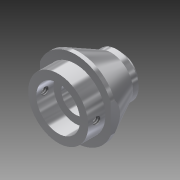
# Autodesk Inventor part: Pneumatic Connector -Actuator Side
Saved by Autodesk Inventor 2013 (Build 170138000, 138)
## iProperties
Created: 2013-06-08
Part Number: Pneumatic Connector -Actuator Side
Material: Generic
Document SubType Name: Modeling
Designer: mvarma
Density: 1 g/cm^3
Author: mvarma
Autodesk Inventor part; units mm, degrees
ref_plane "YZ Plane" through (0, 0, 0) normal (1, 0, 0) x (0, 1, 0)
ref_plane "XZ Plane" through (0, 0, 0) normal (0, 1, 0) x (-1, 0, 0)
ref_plane "XY Plane" through (0, 0, 0) normal (0, 0, 1) x (1, 0, 0)
sketch "Sketch1" plane through (0, 0, 0) normal (0, 0, 1) x (1, 0, 0)
  arc A0 (-1.508, 2.794) -> (-1.508, -2.794) centre (0, 0) ccw
  line L0 (-3.175, 0) -> (0, 0) construction
  line L1 (0, 0) -> (3.175, 0) construction
  line L2 (-1.508, 2.794) -> (1.508, 2.794)
  line L3 (-1.508, -2.794) -> (1.508, -2.794)
  arc A1 (1.508, 2.794) -> (-1.508, 2.794) centre (0, 0) ccw construction
  arc A2 (1.508, -2.794) -> (1.508, 2.794) centre (0, 0) ccw
  arc A3 (-1.508, -2.794) -> (1.508, -2.794) centre (0, 0) ccw construction
  circle A4 centre (0, 0) radius 3.429 construction
  circle A5 centre (0, 0) radius 4.064
  circle A6 centre (0, 0) radius 11.1125
  dimension "d1" = 2.794
  dimension "d2" = 3.175
  dimension "d3" = 6.858
  dimension "d5" = 0.635
  dimension "d6" = 22.225
  constraints: 14 point on circle, 8 end point, 7 centre point, 4 coincident, 2 parallel, 1 collinear, 1 horizontal, 1 other
  measures "d1" distance between parallel lines of L0 L2
  measures "d2" radius of A0
  measures "d3" diameter of A4
  measures "d5" radial gap between concentric circles of A5 A4
  measures "d6" diameter of A6
extrude "Extrusion1" add sketch "Sketch1" along normal blind 3.048 contours A5 | A6
sketch "Sketch2" plane through (0, 0, 3.048) normal (0, 0, 1) x (1, 0, 0)
  circle A0 centre (0, 0) radius 11.1125 projected
  arc A1 (-1.508, 2.794) -> (-1.508, -2.794) centre (0, 0) ccw projected
  constraints: 1 coincident
extrude "Extrusion2" add sketch "Sketch2" along normal blind 3.175
hole "Hole1" at (0, 0, 3.048) direction (0, 0, 1) diameter 3.302 depth 25.4 tip angle 118 thread size "8-32 UNC" class "2B" standard "ANSI Unified Screw Threads"
sketch "Sketch3" plane through (0, 0, 6.223) normal (0, 0, 1) x (1, 0, 0)
  circle A0 centre (0, 0) radius 11.1125 projected
  circle A1 centre (0, 0) radius 3.429
  circle A2 centre (0, 0) radius 4.064
  dimension "d18" = 6.858
  dimension "d19" = 0.635
  constraints: 2 centre point, 2 coincident
  measures "d18" diameter of A1
  measures "d19" radial gap between concentric circles of A2 A1
extrude "Extrusion3" add sketch "Sketch3" along normal blind 7.2961 contours A0
chamfer "Chamfer1" distance 6.35 distance2 12.3571 1 edges at (-11.1125, 0, 0) measured on face at (-10.6125, 0, 0)
sketch "Sketch6" plane through (0, 0, 13.5191) normal (0, 0, 1) x (1, 0, 0)
  circle A0 centre (0, 0) radius 11.1125 projected
  circle A1 centre (0, 0) radius 6.35
  circle A2 centre (0, 0) radius 8.7312
  dimension "d38" = 12.7
  dimension "d52" = 2.3813
  dimension "d53" = 2.3813
  constraints: 2 centre point, 2 coincident
  measures "d38" diameter of A1
  measures "d52" radial gap between concentric circles of A1 A2
  measures "d53" radial gap between concentric circles of A0 A2
extrude "Extrusion5" add sketch "Sketch6" along normal blind 4.9784 contours A2
sketch "Sketch7" plane through (0, 0, 0) normal (1, 0, 0) x (0, 1, 0)
  line L0 (-6.35, 18.4975) -> (6.35, 18.4975) projected
  line L1 (6.35, 13.5191) -> (-6.35, 13.5191) projected
  line L2 (0, 0) -> (0, 13.5191) construction
  line L3 (0, 13.5191) -> (0, 18.4975) construction
  point P0 (0, 16.0084)
  constraints: 4 end point, 3 midpoint, 1 vertical
hole "Hole3" at (0, 0, 16.0084) direction (-1, 0, 0) diameter 2.159 end through all
sketch "Sketch8" plane through (0, 0, 13.5191) normal (0, 0, 1) x (1, 0, 0)
  circle A0 centre (0, 0) radius 11.1125 projected
  circle A1 centre (0, 0) radius 8.7312 projected
  line L0 (-10.3187, 4.1244) -> (-10.3188, -4.1244)
  line L1 (-11.1125, 0) -> (0, 0)
  dimension "d49" = 0.7937
  constraints: 4 end point, 3 point on circle, 1 perpendicular, 1 vertical
  measures "d49" distance from line of L1.start L0
extrude "Extrusion6" cut sketch "Sketch8" against normal through all contours L0 L1 A0 | A0 L1 L0
mirror "Mirror2" about plane through (0, 0, 0) normal (1, 0, 0) of "Hole3", "Extrusion6"
ref_plane "Work Plane3" through (0, 0, 1.4478) normal (0, 0, -1) x (-1, 0, 0)
sketch "Sketch12" plane through (0, 0, 1.4478) normal (0, 0, -1) x (-1, 0, 0)
  circle A0 centre (0, 0) radius 6.35
  circle A1 centre (0, 0) radius 5.0165
  dimension "d60" = 12.7
  dimension "d61" = 10.033
  constraints: 2 centre point, 2 coincident
  measures "d60" diameter of A0
  measures "d61" diameter of A1
extrude "Extrusion9" add sketch "Sketch12" against normal blind 2.54
equation "\"d52\" = d53"
body "Solid1"
